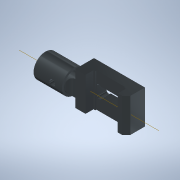
# Autodesk Inventor part: crosse
Saved by Autodesk Inventor 2022.2 (Build 262287000, 287)
## iProperties
Created: 2002-07-03
Part Number: crosse
Material: Acier doux
Document SubType Name: Modélisation
Designer: robert
Density: 7.86 g/cm^3
Appearance: Fonte grise
Control State: 0
Master: False
Checked Out: False
Shininess: 31.0
Length Units: 11269
Angle Units: 11279
Time Units: 11290
Mass Units: 11283
Length Display Precision: 3
Angle Display Precision: 2
Compacted: True
Density: 0.0
Volumn: 0.0
Area: 0.0
PropertySet Name: Model Information
Author: robert
Autodesk Inventor part; units mm, degrees
ref_plane "Plan de construction1" through (90, 28, -30) normal (0, 0, 1) x (1, 0, 0)
sketch "Esquisse1" plane through (90, 28, -30) normal (0, 0, 1) x (1, 0, 0)
  line L0 (0, 0) -> (-90, 0)
  line L1 (0, 0) -> (0, -26)
  line L2 (0, -26) -> (-7, -33)
  line L3 (-7, -33) -> (-15, -33)
  line L4 (-15, -19) -> (-15, -33)
  line L5 (-15, -19) -> (-18, -19)
  line L6 (-69, -17) -> (-18, -17)
  line L7 (-72, -19) -> (-69, -19)
  line L8 (-72, -33) -> (-72, -19)
  line L9 (-90, -33) -> (-72, -33)
  line L10 (-90, -33) -> (-90, 0)
  line L11 (-69, -17) -> (-69, -19)
  line L12 (-18, -17) -> (-18, -19)
  dimension "d10" = 17
  dimension "d11" = 16
  dimension "d12" = 18
  dimension "d13" = 15
  dimension "d14" = 3
  dimension "d15" = 2
  dimension "d17" = 3
  dimension "d18" = 2
  dimension "d19" = 51
  constraints: 26 end point, 2 parallel, 1 collinear
  measures "d10" distance between parallel lines of L6 L0
  measures "d11" distance between parallel lines of L9 L6
  measures "d12" distance between parallel lines of L8 L10
  measures "d13" distance between parallel lines of L1 L4
  measures "d14" distance between parallel lines of L8 L11
  measures "d15" distance between parallel lines of L7 L6
  measures "d17" distance between parallel lines of L4 L12
  measures "d18" distance between parallel lines of L6 L5
  measures "d19" distance between parallel lines of L12 L11
extrude "Extrusion1" add sketch "Esquisse1" along normal blind 60
sketch "Esquisse2" plane through (21, 11, -30) normal (0, -1, 0) x (1, 0, 0)
  line L0 (42.535898, 20.5) -> (8.464102, 20.5)
  line L1 (8.464102, 39.5) -> (42.535898, 39.5)
  arc A0 (50, 37.5) -> (42.535898, 39.5) centre (46, 37.5) ccw
  arc A1 (42.535898, 20.5) -> (50, 22.5) centre (46, 22.5) ccw
  line L2 (50, 37.5) -> (50, 22.5)
  arc A2 (8.464102, 39.5) -> (1, 37.5) centre (5, 37.5) ccw
  line L3 (1, 22.5) -> (1, 37.5)
  arc A3 (1, 22.5) -> (8.464102, 20.5) centre (5, 22.5) ccw
  line L4 (51, 60) -> (0, 60)
  line L5 (0, 0) -> (0, 60)
  line L6 (0, 0) -> (51, 0)
  line L7 (51, 0) -> (51, 60)
  constraints: 16 end point, 8 point on circle, 4 centre point
extrude "Extrusion2" cut sketch "Esquisse2" against normal through all contours L0 A3 L3 A2 L1 A0 L2 A1
ref_plane "Plan de construction2" through (18, -5, 0) normal (0, 0, 1) x (1, 0, 0)
sketch "Esquisse3" plane through (18, -5, 0) normal (0, 0, 1) x (1, 0, 0)
  line L0 (-80, 34) -> (-80, -16)
  line L1 (-42, -7.5) -> (-42, 21.8)
  line L2 (-80, 9) -> (-42, 9)
  line L3 (-42, 9) -> (-42, 21.8)
  line L4 (-42, 21.8) -> (-80, 21.8)
  line L5 (-80, 21.8) -> (-80, 9)
  line L6 (-30, -12) -> (-30, 26)
  line L7 (-80, 9) -> (-30, 9)
  line L8 (-30, 9) -> (-30, -12)
  line L9 (-30, -12) -> (-80, -12)
  line L10 (-80, -12) -> (-80, 9)
  line L11 (-18, 0) -> (-18, 26)
  line L12 (-30, 9) -> (-18, 9)
  line L13 (-18, 9) -> (-18, 26)
  line L14 (-18, 26) -> (-30, 26)
  line L15 (-30, 26) -> (-30, 9)
  line L16 (0, 14) -> (0, 0)
  line L17 (0, 7) -> (-22.134302, 7)
  line L18 (-18, 0) -> (-18, 33)
  dimension "d20" = 21
  dimension "d21" = 12.8
  dimension "d22" = 12
  dimension "d23" = 62
  dimension "d24" = 17
  dimension "d29" = 2
  dimension "d30" = 38
  constraints: 34 end point, 6 parallel, 4 perpendicular, 3 horizontal, 2 collinear, 2 midpoint
  measures "d20" distance between parallel lines of L9 L7
  measures "d21" distance between parallel lines of L4 L2
  measures "d22" distance between parallel lines of L11 L15
  measures "d23" distance between parallel lines of L0 L11
  measures "d24" distance between parallel lines of L14 L12
  measures "d29" distance between parallel lines of L12 L17
  measures "d30" distance between parallel lines of L0 L1
revolve "Révolution1" add sketch "Esquisse3" angle 360 about axis through (-62, 4, 0) along (1, 0, 0) contours L6 L14 L11 L12 | L2 L7 L6 L9 L0
revolve "Révolution2" cut sketch "Esquisse3" angle 360 about axis through (-62, 4, 0) along (1, 0, 0) contours L4 L1 L2 L0
sketch "Esquisse5" plane through (18, -5, 0) normal (0, 0, 1) x (1, 0, 0)
  arc A0 (-18, 0) -> (-30, -12) centre (-18, -12) ccw
  line L0 (-18, 0) -> (-18, 0)
  line L1 (-30, 9) -> (-18, 9) projected
  line L2 (-18, -8) -> (-18, 0) projected
  line L3 (-18, -12) -> (-30, -12)
  line L4 (-18, 0) -> (0, 0) projected
  line L5 (-30, -8) -> (-30, 26) projected
  dimension "d31" = 12
  constraints: 4 end point, 2 point on circle, 2 tangent, 1 centre point, 1 collinear, 1 parallel, 1 perpendicular, 1 point on line
  measures "d31" radius of A0
sketch "Esquisse5 outline for Extrusion3" plane through (18, -5, 0) normal (0, 0, 1) x (1, 0, 0)
  arc A0 (-18, 0) -> (-30, -12) centre (-18, -12) ccw
  line L0 (-18, -8) -> (-18, 0)
  line L1 (-30, -12) -> (-18, -8)
extrude "Extrusion3" cut sketch "Esquisse5 outline for Extrusion3" along normal through all both and the other way through all
ref_plane "Plan de construction3" through (-37, 4, 0) normal (0, -1, 0) x (1, 0, 0)
sketch "Esquisse6" plane through (-37, 4, 0) normal (0, -1, 0) x (1, 0, 0)
  arc A0 (5.953227, 4.562013) -> (11.578201, 3.492329) centre (7.999875, -0.000026) ccw
  circle A1 centre (7.999875, -0.000026) radius 5.000096
  dimension "d26" = 5.0001
  constraints: 2 centre point, 2 point on circle, 1 coincident, 1 concentric
  measures "d26" radius of A0
extrude "Extrusion4" cut sketch "Esquisse6" along normal through all
sketch "Esquisse7" plane through (-24, 4, 0) normal (-1, 0, 0) x (0, 0, 1)
  circle A0 centre (0, 0) radius 12.8 projected
  constraints: 1 coincident
hole "Perçage1" at (-24, 4, 0) direction (1, 0, 0) diameter 4.134 depth 19.5 tip angle 118 counterbore diameter 8 counterbore depth 4.5 thread size "M5x0.8" class "6H" standard "ISO Metric profile"
sketch "Esquisse8" plane through (-24, 4, 0) normal (-1, 0, 0) x (0, 0, 1)
  circle A0 centre (0, 0) radius 4 projected
  circle A1 centre (0, 0) radius 12.8 projected
  line L0 (-12.8, 0) -> (12.8, 0)
  constraints: 2 end point, 2 point on circle, 1 horizontal
